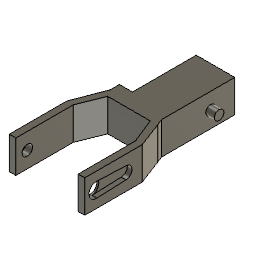
Elbow (Autodesk Fusion 360 design; units mm, degrees)
part number: 2026-08-08-17-19-53-385
Autodesk Fusion 360 part; units mm, degrees
sketch "Sketch1" plane through (0, 0, 0) normal (0, 0, 1) x (1, 0, 0)
  line L0 (-16.25, -0.6886) -> (-16.25, 29.3114)
  line L1 (-16.25, 29.3114) -> (-19.75, 29.3114)
  line L2 (-19.75, 29.3114) -> (-19.75, -0.6886)
  line L3 (-19.75, -0.6886) -> (-16.25, -0.6886)
  spline S0 degree 3 poles (-19.7481, 22.9091) (-19.7487, 22.9276) (-19.7494, 22.9461) (-19.75, 22.9645) knots 0 0 0 0 0.001755 0.001755 0.001755 0.001755
  line L4 (-16.25, 29.3114) -> (-11.1067, 42.1478)
  line L5 (-11.1067, 42.1478) -> (0, 42.1478)
  line L6 (0, 42.1478) -> (0, 45.6478)
  line L7 (-14.7933, 42.3572) -> (-13.4749, 45.6478)
  line L8 (-13.4749, 45.6478) -> (0, 45.6478)
  line L9 (-19.75, 29.3114) -> (-14.7933, 42.3572)
  dimension "d1" = 3.5
  dimension "d2" = 16.25
  dimension "d3" = 30
  dimension "d8" = -3.5
  constraint vertical L0
  constraint perpendicular L0 L1
  constraint perpendicular L1 L2
  constraint perpendicular L0 L3
  constraint coincident L2 S0.end
  constraint perpendicular L0 L5
  constraint perpendicular L5 L6
  measures "d1" distance of L0.start L2.end
  measures "d2" distance of origin L0
  measures "d3" distance of L0.start L0.end
extrude "Extrude1" add sketch "Sketch1" along normal blind 12 contours L0 L1 L2 L3 S0
extrude "Extrude2" add sketch "Sketch1" along normal blind 17
mirror "Mirror1" about plane through (0, 0, 0) normal (1, 0, 0) of bodies 1 merged
sketch "Sketch2" plane through (19.75, 0, 0) normal (1, 0, 0) x (0, 1, 0)
  line L0 (-0.6886, 0) -> (29.3114, 0)
  line L1 (29.3114, 0) -> (29.3114, 17)
  line L2 (29.3114, 17) -> (-0.6886, 17)
  line L3 (-0.6886, 17) -> (-0.6886, 0)
  line L4 (-0.6886, 8.5) -> (29.3114, 8.5) construction
  line L5 (23.3114, 9.6158) -> (23.3114, 7.3842) construction
  line L6 (5.3214, 12.3) -> (5.8374, 12.2634)
  circle A0 centre (5.3114, 8.5) radius 3.8
  arc A1 (20.7878, 5.3) -> (20.9673, 11.695) centre (20.7889, 8.5) ccw
  line L7 (20.9673, 11.695) -> (5.3214, 12.3)
  line L8 (20.7878, 5.3) -> (5.3209, 4.7)
  point P0 (9.3621, 0)
  point P1 (23.3114, 8.5)
  point P2 (6.3843, 8.5)
  dimension "d31" = 6
  dimension "d32" = 18
  dimension "d40" = 7.6
  dimension "d45" = 3.2
  constraint coincident L0 P0
  constraint midpoint L3 L4.start
  constraint midpoint L1 L4.end
  constraint midpoint L5 P1
  constraint coincident L4 P1
  constraint perpendicular L4 L5
  constraint coincident L4 P2
  constraint coincident A0 L6.start
  constraint coincident L4 A1.centre
  constraint coincident L6.end A0
  constraint coincident L8.end A0
  constraint coincident L4 A0.centre
  measures "d31" distance of L3 A0.centre
  measures "d32" distance of L5 A0.centre
  measures "d40" diameter of A0
  measures "d45" radius of A1
sketch "Sketch4" plane through (0, 42.1478, 0) normal (0, -1, 0) x (1, 0, 0)
  line L0 (-11.1067, 0) -> (11.1067, 0)
  line L1 (11.1067, 0) -> (11.1067, 17)
  line L2 (11.1067, 17) -> (-11.1067, 17)
  line L3 (-11.1067, 17) -> (-11.1067, 0)
sketch "Sketch5" plane through (0, 45.6478, 0) normal (0, 1, 0) x (-1, 0, 0)
  line L0 (-13.4749, 0) -> (13.4749, 0)
  line L1 (13.4749, 0) -> (13.4749, 17)
  line L2 (13.4749, 17) -> (-13.4749, 17)
  line L3 (-13.4749, 17) -> (-13.4749, 0)
extrude "Extrude7" cut sketch "Sketch2" against normal blind 1.5 from surface at -2 contours L6 A0 L7 | L6 A0 L8
extrude "Extrude8" cut sketch "Sketch2" against normal blind 4 contours L6 A0 L7 | L6 A0 L8 | A0 L7 | A0 L8
extrude "Extrude9" cut sketch "Sketch2" against normal blind 2.5 contours A0 A1 L7 L8
sketch "Sketch6" plane through (-19.75, 0, 0) normal (-1, 0, 0) x (0, -1, 0)
  line L0 (-29.3114, 0) -> (0.6886, 0)
  line L1 (0.6886, 0) -> (0.6886, 17)
  line L2 (0.6886, 17) -> (-29.3114, 17)
  line L3 (-29.3114, 17) -> (-29.3114, 0)
  circle A0 centre (-5.3114, 8.5) radius 2.75
  line L4 (-29.3114, 0) -> (0.6886, 0)
  point P0 (0.6886, 8.5)
  dimension "d49" = 5.5
  dimension "d52" = 6
  dimension "d53" = 8.5
  measures "d49" diameter of A0
  measures "d52" horizontal distance of A0.centre P0
  measures "d53" distance of A0.centre L4
extrude "Extrude10" cut sketch "Sketch6" against normal blind 4 contours A0
extrude "Extrude11" add sketch "Sketch5" along normal blind 5
sketch "Sketch7" plane through (0, 50.6478, 0) normal (0, 1, 0) x (-1, 0, 0)
  line L0 (-13.4749, 17) -> (-13.4749, 0)
  line L1 (-13.4749, 0) -> (13.4749, 0)
  line L2 (13.4749, 0) -> (13.4749, 17)
  line L3 (13.4749, 17) -> (-13.4749, 17)
  line L4 (-10.9749, 2.25) -> (6.6749, 2.25) construction
  line L5 (13.4749, 0) -> (0, 0) construction
  line L6 (6.6751, 14.75) -> (-10.9749, 14.75)
  line L7 (-10.9749, 14.75) -> (-10.9749, 2.25)
  line L8 (-10.9749, 2.25) -> (6.6749, 2.25)
  line L9 (6.6751, 14.75) -> (6.6751, 17)
  line L10 (6.6749, 2.25) -> (6.7374, 0)
  line L11 (6.6749, 14.75) -> (6.6749, 2.25)
  point P0 (-2.15, 2.25)
  point P1 (13.4749, 0)
  point P2 (6.6749, 8.5)
  point P3 (6.6749, 8.5)
  dimension "d57" = 2.25
  dimension "d61" = 2.25
  dimension "d73" = 12.5
  dimension "d74" = 17.65
  constraint midpoint L4 P0
  constraint perpendicular L0 L4
  constraint coincident L4 L8.end
  constraint coincident L3 L9.end
  constraint perpendicular L3 L9
  constraint midpoint L5 L10.end
  constraint midpoint L11 P3
  constraint coincident P3 P2
  constraint perpendicular L8 L11
  measures "d57" distance of L4 L5
  measures "d61" distance of L3 L6
  measures "d73" distance of L4.start L6.end
  measures "d74" distance of L6.start L6.end
extrude "Extrude12" add sketch "Sketch7" along normal blind 4.9 contours L6 L7 L8 L11
sketch "Sketch8" plane through (-6.6749, 0, 0) normal (-1, 0, 0) x (0, -1, 0)
  line L0 (-50.6478, 2.5) -> (-50.6478, 14.5)
  line L1 (-50.6478, 14.5) -> (-55.5478, 14.5)
  line L2 (-55.5478, 14.5) -> (-55.5478, 2.5)
  line L3 (-55.5478, 2.5) -> (-50.6478, 2.5)
  line L4 (-53.0978, 14.5) -> (-53.0978, 2.5) construction
  circle A0 centre (-53.0978, 8.5) radius 0.9
  line L5 (-50.6478, 2.25) -> (-50.6478, 14.75)
  line L6 (-50.6478, 14.75) -> (-55.5478, 14.75)
  line L7 (-55.5478, 14.75) -> (-55.5478, 2.25)
  line L8 (-55.5478, 2.25) -> (-50.6478, 2.25)
  dimension "d66" = 1.8
  constraint coincident L1 L4.start
  constraint coincident L3 L4.end
  constraint perpendicular L3 L4
  constraint midpoint L4 A0.centre
  measures "d66" diameter of A0
extrude "Extrude13" cut sketch "Sketch8" against normal blind 8 contours A0
extrude "Extrude14" add sketch "Sketch7" along normal blind 33.3 contours L0 L1 L3 L6 L7 L8 L9 L10
ref_plane "WorkPlane1" through (2.15, 67.2978, 8.5) normal (0, 1, 0) x (0, 0, 1)
mirror "Mirror2" about plane through (2.15, 67.2978, 8.5) normal (0, 1, 0) of "Extrude12", "Extrude13"
sketch "Sketch10" plane through (10.9749, 0, 0) normal (-1, 0, 0) x (0, -1, 0)
  line L0 (-79.0478, 14.75) -> (-79.0478, 2.25)
  line L1 (-79.0478, 2.25) -> (-55.5478, 2.25)
  line L2 (-55.5478, 2.25) -> (-55.5478, 14.75)
  line L3 (-55.5478, 14.75) -> (-79.0478, 14.75)
  line L4 (-71.2478, 14.75) -> (-71.2478, 2.25) construction
  circle A0 centre (-71.2478, 8.5) radius 2.5
  point P0 (-50.6478, 8.5)
  dimension "d81" = 5
  dimension "d84" = 20.6
  constraint coincident L3 L4.start
  constraint coincident L1 L4.end
  constraint perpendicular L1 L4
  constraint midpoint L4 A0.centre
  measures "d81" diameter of A0
  measures "d84" distance of A0.centre P0
extrude "Extrude15" add sketch "Sketch10" against normal blind 7 contours A0
sketch "Sketch11" plane through (0, 83.9478, 0) normal (0, 1, 0) x (-1, 0, 0)
  line L0 (6.6751, 14.75) -> (6.6751, 17)
  line L1 (6.6751, 17) -> (-13.4749, 17)
  line L2 (-13.4749, 17) -> (-13.4749, 0)
  line L3 (-13.4749, 0) -> (6.7374, 0)
  line L4 (6.7374, 0) -> (6.6749, 2.25)
  line L5 (6.6749, 2.25) -> (6.6749, 14.75)
  line L6 (6.6749, 14.75) -> (6.6751, 14.75)
  line L7 (-11.0192, 14.7733) -> (6.6749, 14.7733)
  line L8 (6.6749, 14.7733) -> (6.6749, 14.75)
  line L9 (-9.9749, 13.25) -> (-5.4749, 13.25)
  line L10 (-5.4749, 13.25) -> (-5.4749, 4.25)
  line L11 (-5.4749, 4.25) -> (-9.9749, 4.25)
  line L12 (-9.9749, 4.25) -> (-9.9749, 13.25)
  dimension "d86" = 4.5
  dimension "d87" = 3.5
  dimension "d89" = 3.75
  dimension "d90" = 9
  constraint horizontal L7
  constraint vertical L8
  constraint horizontal L9
  constraint vertical L10
  constraint horizontal L11
  constraint vertical L12
  measures "d86" distance of L10.end L11.end
  measures "d87" distance of L2 L12
  measures "d89" distance of L1 L9
  measures "d90" distance of L9.end L10.end
extrude "Extrude16" cut sketch "Sketch11" against normal blind 5 contours L9 L10 L11 L12
move_face "OffsetFaces1" offset -0.25 6 faces at (5.0916, 63.3811, 2.25) (-2.625, 79.0478, 7.0833) (10.9749, 71.2804, 8.0846) (10.9749, 59.9478, 8.5) (-0.7918, 63.3811, 14.75) (-0.7917, 55.5478, 10.5833)
